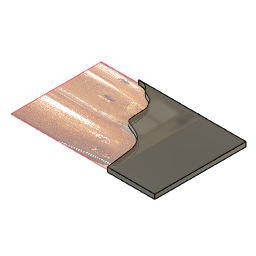
Jack Version 2 v2 (Autodesk Fusion 360 design; units mm, degrees)
Autodesk Fusion 360 part; units mm, degrees
sketch "Sketch6" plane through (0, 0, 0) normal (0, 0, 1) x (1, 0, 0)
  spline S0 degree 5 poles (-21.7729, 19.496) (-21.243, 19.4854) (-20.1991, 19.466) (-18.681, 19.4424) (-16.7525, 19.4221) (-14.502, 19.4148) (-12.4129, 19.424) (-10.4865, 19.4462) (-8.724, 19.4759) (-7.1265, 19.5042) (-5.6949, 19.5189) (-4.429, 19.5035) (-3.3282, 19.4363) (-2.3902, 19.2906) (-1.6064, 19.0432) (-0.9567, 18.6813) (-0.4058, 18.21) (0.1041, 17.6624) (0.6407, 17.0876) (1.2636, 16.5339) (2.01, 16.0344) (2.8747, 15.5886) (3.8183, 15.1724) (4.76, 14.7404) (5.6097, 14.2499) (6.2035, 13.6312) (6.5592, 12.9359) (6.8205, 12.278) (7.1339, 11.7469) (7.5184, 11.2993) (7.8624, 10.7732) (8.0408, 10.0025) (8.0849, 8.9911) (8.1008, 7.8284) (8.1298, 6.5443) (8.208, 5.1688) (8.3204, 4.0037) (8.4354, 3.096) (8.5257, 2.4757) (8.5742, 2.1618) knots 0 0 0 0 0 0 0.028571 0.057143 0.085714 0.114286 0.142857 0.171429 0.2 0.228571 0.257143 0.285714 0.314286 0.342857 0.371429 0.4 0.428571 0.457143 0.485714 0.514286 0.542857 0.571429 0.6 0.628571 0.657143 0.685714 0.714286 0.742857 0.771429 0.8 0.828571 0.857143 0.885714 0.914286 0.942857 0.971429 1 1 1 1 1 1
  line L0 (7.4749, 13.6643) -> (8.5251, 6.3357)
  line L1 (1.503, 17.0407) -> (9.2617, 11.6391)
  spline S1 degree 5 poles (8.5742, 2.1618) (8.5541, 2.0883) (8.5433, 1.941) (8.6149, 1.7192) (8.8874, 1.4219) (9.5209, 1.044) (10.4256, 0.649) (11.5488, 0.2153) (12.8193, -0.2847) (14.1567, -0.8816) (15.4811, -1.605) (16.7222, -2.4799) (17.83, -3.5211) (18.7762, -4.7336) (19.5464, -6.1166) (20.1362, -7.6662) (20.4644, -9.0352) (20.6313, -10.1329) (20.7075, -10.896) (20.7368, -11.2853) knots 0 0 0 0 0 0 0.066667 0.133333 0.2 0.266667 0.333333 0.4 0.466667 0.533333 0.6 0.666667 0.733333 0.8 0.866667 0.933333 1 1 1 1 1 1
  line L2 (-21.7729, 19.496) -> (43, 19.496)
  line L3 (43, 19.496) -> (43, -24)
  spline S2 degree 5 poles (20.7368, -11.2853) (20.7873, -11.6739) (20.8884, -12.4511) (21.04, -13.6169) (21.2421, -15.1712) (21.4947, -17.1141) (21.6968, -18.6685) (21.8484, -19.8342) (21.9495, -20.6114) (22, -21) knots 0 0 0 0 0 0 0.2 0.4 0.6 0.8 1 1 1 1 1 1
  line L4 (22, -21) -> (43, -21)
  point P0 (-4.6352, 19.496)
  point P1 (-0.854, 18.563)
  point P2 (1.3557, 16.5006)
  point P3 (5.3824, 14.3399)
  point P4 (7, 12)
  point P5 (8, 10)
  point P6 (9.5072, 1.0815)
  point P7 (16, -2)
  constraint midpoint P5 L0
  constraint midpoint P3 L1
  constraint horizontal L2
  constraint perpendicular L2 L3
  constraint coincident L3 L4.end
  constraint perpendicular L3 L4
extrude "Extrude1" add sketch "Sketch6" along normal blind 2 contours S0 L0 L1 S1 L2 L3 S2 L4 | S0 L0 L1
